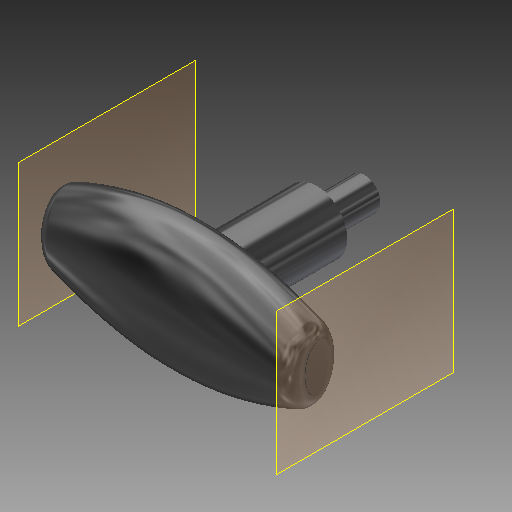
# Autodesk Inventor part: Starter Handle
Saved by Autodesk Inventor 2017 (Build 210142000, 142)
## iProperties
Created: 2012-09-28
Part Number: Starter Handle
Material: Rubber
Document SubType Name: Modeling
Designer: John
Density: 1 g/cm^3
Appearance: Rubber - Black - Version 1.1
Author: John
Autodesk Inventor part; units mm, degrees
ref_plane "XZ Plane" through (0, 0, 0) normal (0, 1, 0) x (-1, 0, 0)
ref_plane "XY Plane" through (0, 0, 0) normal (0, 0, 1) x (1, 0, 0)
sketch "Sketch1" plane through (0, 0, 0) normal (0, 0, 1) x (1, 0, 0)
  circle A0 centre (0, 0) radius 3.048
  dimension "d0" = 6.096
  constraints: 1 centre point, 1 coincident
  measures "d0" diameter of A0
extrude "Extrusion1" add sketch "Sketch1" along normal blind 12.7
sketch "Sketch2" plane through (0, 0, 0) normal (1, 0, 0) x (0, 1, 0)
  line L0 (3.048, 12.7) -> (3.048, 0) projected
  line L1 (3.048, 0) -> (-3.048, 0) projected
  line L2 (-3.048, 0) -> (-3.048, 12.7) projected
  line L3 (-3.048, 12.7) -> (3.048, 12.7) projected
  ellipse E0 centre (0, 12.7) end of major axis (6.35, 12.7) minor radius 3.175
  point P0 (0, 0)
  dimension "d4" = 6.35
  dimension "d6" = 3.175
  constraints: 1 midpoint, 2 other
ref_plane "Work Plane1" through (12.7, 0, 0) normal (1, 0, 0) x (0, 1, 0)
ref_plane "Work Plane2" through (-12.7, 0, 0) normal (1, 0, 0) x (0, 1, 0)
sketch "Sketch3" plane through (12.7, 0, 0) normal (1, 0, 0) x (0, 1, 0)
  line L0 (3.048, 12.7) -> (-3.048, 12.7) projected
  ellipse E0 centre (0, 12.7) end of major axis (3.175, 12.7) minor radius 2.54
  point P0 (0, 0)
  dimension "d9" = 3.175
  dimension "d13" = 2.54
  constraints: 1 midpoint, 2 other
sketch "Sketch4" plane through (-12.7, 0, 0) normal (1, 0, 0) x (0, 1, 0)
  ellipse E0 centre (0, 12.7) end of major axis (3.175, 12.7) minor radius 2.54 projected
  point P0 (0, 0)
  constraints: 1 other
sketch "Sketch3 outline for Loft1" plane through (12.7, 0, 0) normal (1, 0, 0) x (0, 1, 0)
  spline S0 degree 2 poles (3.175, 12.7) (3.175, 17.099409) (-1.5875, 14.899705) (-6.35, 12.7) (-1.5875, 10.500295) (3.175, 8.300591) (3.175, 12.7) knots 0 0 0 0.33333333 0.33333333 0.66666667 0.66666667 1 1 1 weights 1 0.5 1 0.5 1 0.5 1
sketch "Sketch2 outline for Loft1" plane through (0, 0, 0) normal (1, 0, 0) x (0, 1, 0)
  spline S0 degree 2 poles (6.35, 12.7) (6.35, 18.199261) (-3.175, 15.449631) (-12.7, 12.7) (-3.175, 9.950369) (6.35, 7.200739) (6.35, 12.7) knots 0 0 0 0.33333333 0.33333333 0.66666667 0.66666667 1 1 1 weights 1 0.5 1 0.5 1 0.5 1
sketch "Sketch4 outline for Loft1" plane through (-12.7, 0, 0) normal (1, 0, 0) x (0, 1, 0)
  spline S0 degree 2 poles (3.175, 12.7) (3.175, 17.099409) (-1.5875, 14.899705) (-6.35, 12.7) (-1.5875, 10.500295) (3.175, 8.300591) (3.175, 12.7) knots 0 0 0 0.33333333 0.33333333 0.66666667 0.66666667 1 1 1 weights 1 0.5 1 0.5 1 0.5 1
loft "Loft1" add profiles "Sketch3 outline for Loft1", "Sketch2 outline for Loft1", "Sketch4 outline for Loft1"
fillet "Fillet1" radius 1.5875 4 edges at (3.0466, -0.0909, 9.5619) (-3.0465, 0.095, 9.5619) (12.7, -3.175, 12.7) (-12.7, -3.175, 12.7)
sketch "Sketch5" plane through (0, 0, 0) normal (0, 0, -1) x (-1, 0, 0)
  circle A0 centre (0, 0) radius 3.048 projected
  circle A1 centre (0, 0) radius 1.5748
  dimension "d21" = 3.1496
  constraints: 1 centre point, 1 coincident
  measures "d21" diameter of A1
extrude "Extrusion2" add sketch "Sketch5" along normal blind 4.7625 contours A1
body "Solid1"
